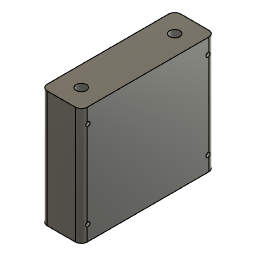
VibrometerPositioningTable v34 (Autodesk Fusion 360 archive; units mm, degrees)
design "Base Spacer"
Autodesk Fusion 360 part; units mm, degrees
sketch "Sketch1" plane through (0, 0, 0) normal (0, 1, 0) x (1, 0, 0)
  line L0 (-12, 40) -> (12, 40)
  line L1 (12, 40) -> (12, -40)
  line L2 (12, -40) -> (-12, -40)
  line L3 (-12, -40) -> (-12, 40)
  line L4 (-50, 0) -> (40, 0) construction
  line L5 (0, 60) -> (0, -56.3927) construction
  circle A0 centre (0, -28) radius 3.1
  circle A1 centre (0, 28) radius 3.1
  dimension "d1" = 24
  dimension "d2" = 80
  dimension "d3" = 12
  dimension "d4" = 40
  dimension "d5" = 6.2
  dimension "d6" = 12
  dimension "d7" = 12
  constraint horizontal L0
  constraint vertical L1
  constraint horizontal L2
  constraint vertical L3
  constraint horizontal L4
  constraint perpendicular L2 L5
  constraint symmetric L4 A0 A1
  measures "d1" distance of L0.start L0.end
  measures "d2" distance of L0.start L2.end
  measures "d3" distance of L3 L5
  measures "d4" distance of L0 L4
  measures "d5" diameter of A0
  measures "d6" distance of L3 A0.centre
  measures "d7" distance of L2 A0.centre
extrude "Extrude1" add sketch "Sketch1" along normal blind 70
fillet "Fillet1" radius 3.5 4 edges at (-12, 35, 40) (-12, 35, -40) (12, 35, -40) (12, 35, 40)
sketch "Sketch3" plane through (12, 0, 0) normal (1, 0, 0) x (0, 0, -1)
  line L0 (-36.5, 70) -> (-36.5, 0)
  line L1 (-36.5, 0) -> (36.5, 0)
  line L2 (36.5, 0) -> (36.5, 70)
  line L3 (36.5, 70) -> (-36.5, 70)
  line L4 (36, 9) -> (-36, 9)
  line L5 (-36, 9) -> (-36, 61)
  line L6 (-36, 61) -> (36, 61)
  line L7 (36, 61) -> (36, 9)
  line L8 (36, 9) -> (-36, 61) construction
  line L9 (-36, 9) -> (36, 61) construction
  circle A0 centre (-36, 61) radius 1.25
  circle A1 centre (36, 61) radius 1.25
  circle A2 centre (-36, 9) radius 1.25
  circle A3 centre (36, 9) radius 1.25
  point P0 (0, 35)
  dimension "d12" = 72
  dimension "d13" = 52
  dimension "d14" = 36.5
  dimension "d15" = 73
  dimension "d16" = 2.5
  dimension "d17" = 2.5
  dimension "d18" = 2.5
  dimension "d19" = 2.5
  dimension "d20" = 70
  dimension "d21" = 35
  constraint horizontal L4
  constraint perpendicular L4 L5
  constraint parallel L4 L6
  constraint parallel L5 L7
  constraint coincident L8 P0
  constraint coincident L9 P0
  constraint coincident L5.end L6.start
  constraint coincident L6.end L7.start
  constraint coincident L4.end L5.start
  constraint coincident L4.start L7.end
  measures "d12" distance of L5.end L6.end
  measures "d13" distance of L4.end L5.end
  measures "d14" distance of L0 P0
  measures "d15" distance of L0.start L2.end
  measures "d16" diameter of A0
  measures "d17" diameter of A1
  measures "d18" diameter of A2
  measures "d19" diameter of A3
  measures "d20" distance of L1 L3
  measures "d21" distance of L3 P0
extrude "Extrude2" cut sketch "Sketch3" against normal blind 24 contours L0 L5 L6 A0 | L0 A0 | L5 L6 A0 | L2 A1 | L2 L6 L7 A1 | L0 L4 L5 A2 | L0 A2 | L6 L7 A1 | L4 L5 A2 | L2 A3 | L2 L4 L7 A3 | L4 L7 A3
equation "d3 = d1 / 2"
equation "d4 = d2 / 2"
equation "d7 = d6"
equation "d14 = d15 / 2"
equation "d17 = d16"
equation "d18 = d16"
equation "d19 = d16"
equation "d21 = d20 / 2"

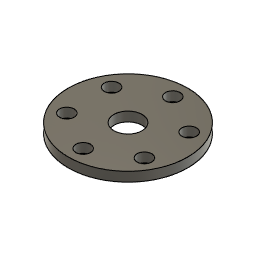
design "HubSpacer2"
Autodesk Fusion 360 part; units mm, degrees
sketch "Sketch1" plane through (0, 0, 0) normal (0, 1, 0) x (1, 0, 0)
  circle A0 centre (0, 0) radius 12.7
  circle A1 centre (0, 0) radius 9.525 construction
  circle A2 centre (-0.0005, 9.525) radius 1.55
  circle A3 centre (-8.2491, 4.7621) radius 1.55
  circle A4 centre (-8.2487, -4.7629) radius 1.55
  circle A5 centre (0.0005, -9.525) radius 1.55
  circle A6 centre (8.2491, -4.7621) radius 1.55
  circle A7 centre (8.2487, 4.7629) radius 1.55
  circle A8 centre (0, 0) radius 3
  dimension "d1" = 25.4
  dimension "d2" = 19.05
  dimension "d3" = 3.1
  dimension "d5" = 360
  dimension "d6" = 6
  constraint coincident A0.centre A1.centre
  constraint concentric A0 A1
  constraint coincident A1 A2.centre
  measures "d1" diameter of A0
  measures "d2" diameter of A1
  measures "d3" diameter of A2
  measures "d6" diameter of A8
extrude "Extrude1" add sketch "Sketch1" along normal blind 2

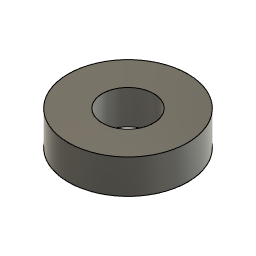
design "BallBearing12x28x8"
Autodesk Fusion 360 part; units mm, degrees
sketch "Sketch1" plane through (0, 0, 0) normal (0, 1, 0) x (1, 0, 0)
  circle A0 centre (0, 0) radius 6
  circle A1 centre (0, 0) radius 14
  dimension "d1" = 12
  dimension "d2" = 28
  constraint coincident A0.centre A1.centre
  constraint concentric A0 A1
  measures "d1" diameter of A0
  measures "d2" diameter of A1
extrude "Extrude1" add sketch "Sketch1" along normal blind 8

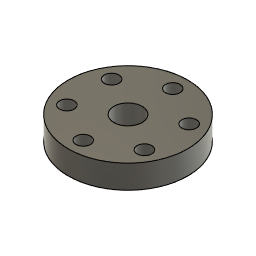
design "HubSpacer5"
Autodesk Fusion 360 part; units mm, degrees
sketch "Sketch1" plane through (0, 0, 0) normal (0, 1, 0) x (1, 0, 0)
  circle A0 centre (0, 0) radius 12.7
  circle A1 centre (0, 0) radius 9.525 construction
  circle A2 centre (-0.0005, 9.525) radius 1.55
  circle A3 centre (-8.2491, 4.7621) radius 1.55
  circle A4 centre (-8.2487, -4.7629) radius 1.55
  circle A5 centre (0.0005, -9.525) radius 1.55
  circle A6 centre (8.2491, -4.7621) radius 1.55
  circle A7 centre (8.2487, 4.7629) radius 1.55
  circle A8 centre (0, 0) radius 3
  dimension "d1" = 25.4
  dimension "d2" = 19.05
  dimension "d3" = 3.1
  dimension "d5" = 360
  dimension "d6" = 6
  constraint coincident A0.centre A1.centre
  constraint concentric A0 A1
  constraint coincident A1 A2.centre
  measures "d1" diameter of A0
  measures "d2" diameter of A1
  measures "d3" diameter of A2
  measures "d6" diameter of A8
extrude "Extrude1" add sketch "Sketch1" along normal blind 5

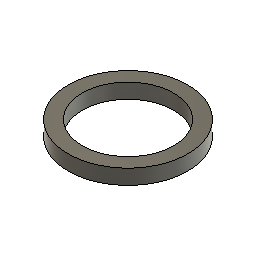
design "BallBearing55x72x9"
Autodesk Fusion 360 part; units mm, degrees
sketch "Sketch1" plane through (0, 0, 0) normal (0, 1, 0) x (1, 0, 0)
  circle A0 centre (0, 0) radius 27.5
  circle A1 centre (0, 0) radius 36
  dimension "d1" = 55
  dimension "d2" = 72
  constraint coincident A0.centre A1.centre
  constraint concentric A0 A1
  measures "d1" diameter of A0
  measures "d2" diameter of A1
extrude "Extrude1" add sketch "Sketch1" along normal blind 9

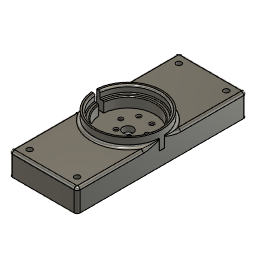
design "StaticBase"
Autodesk Fusion 360 part; units mm, degrees
sketch "Sketch1" plane through (0, 0, 0) normal (0, 1, 0) x (-1, 0, 0)
  circle A0 centre (7.75, 53.037581) radius 1.5
  circle A1 centre (7.75, 26.190794) radius 1.5
  circle A2 centre (-15.5, 39.614187) radius 1.5
  circle A3 centre (-7.75, 26.190794) radius 1.5
  circle A4 centre (15.5, 39.614187) radius 1.5
  circle A5 centre (-7.75, 53.037581) radius 1.5
  circle A6 centre (0, 46.614187) radius 6
  circle A7 centre (-15.5, 39.614187) radius 1.6
  circle A8 centre (-7.75, 53.037581) radius 1.6
  circle A9 centre (7.75, 53.037581) radius 1.6
  circle A10 centre (15.5, 39.614187) radius 1.6
  circle A11 centre (7.75, 26.190794) radius 1.6
  circle A12 centre (-7.75, 26.190794) radius 1.6
  circle A13 centre (0, 46.614187) radius 6.15
  line L0 (40, 39.614187) -> (40, 146.614187)
  line L1 (-40, 39.614187) -> (-40, 146.614187)
  line L2 (-40, 39.614187) -> (-40, -53.385813)
  line L3 (-40, -53.385813) -> (40, -53.385813)
  line L4 (40, -53.385813) -> (40, 39.614187)
  line L5 (40, 146.614187) -> (-40, 146.614187)
  line L6 (40, -13.385813) -> (-40, -13.385813)
  line L7 (40, 106.614187) -> (-40, 106.614187)
  line L8 (0, 150) -> (0, -80) construction
  line L9 (46.540026, 46.614187) -> (-48.931314, 46.614187) construction
  circle A14 centre (0, 39.614187) radius 15.5
  line L10 (35, -13.385813) -> (35, 106.614187)
  line L11 (-35, -13.385813) -> (-35, 106.614187)
  dimension "d24" = 40
  dimension "d25" = 40
  dimension "d5" = 100
  dimension "d6" = 100
  dimension "d11" = 12.3
  dimension "d12" = 3.2
  dimension "d13" = 3.2
  dimension "d14" = 3.2
  dimension "d15" = 3.2
  dimension "d16" = 3.2
  dimension "d17" = 3.2
  dimension "d18" = 15.5
  dimension "d19" = 7
  dimension "d28" = 31
  dimension "d29" = 7
  dimension "d31" = 40
  dimension "d32" = 40
  dimension "d35" = 5
  dimension "d36" = 5
  constraint concentric A5 A8
  constraint concentric A0 A9
  constraint concentric A1 A11
  constraint concentric A3 A12
  constraint concentric A6 A13
  constraint vertical L0
  constraint vertical L1
  constraint perpendicular L0 L3
  constraint perpendicular L3 L4
  constraint perpendicular L0 L5
  constraint perpendicular L2 L6
  constraint perpendicular L1 L7
  constraint perpendicular L5 L8
  constraint perpendicular L1 L9
  constraint symmetric A7 A10 L8
  constraint perpendicular L7 L10
  constraint perpendicular L7 L11
  measures "d24" distance of L3 L6
  measures "d25" distance of L5 L7
  measures "d5" distance of L3 L9
  measures "d6" distance of L5 L9
  measures "d11" diameter of A13
  measures "d12" diameter of A9
  measures "d13" diameter of A10
  measures "d14" diameter of A11
  measures "d15" diameter of A12
  measures "d16" diameter of A7
  measures "d17" diameter of A8
  measures "d28" diameter of A14
  measures "d31" distance of L4 L8
  measures "d32" distance of L2 L8
  measures "d35" distance of L0 L10
  measures "d36" distance of L1 L11
extrude "Extrude7" add sketch "Sketch1" along normal blind 6.5 contours A7 A8 A9 A10 A11 A12 A14 | L0 L4 L6 L7 L10 | L0 L1 L5 L7 | L2 L3 L4 L6 | L6 L7 L10 L11 | L1 L2 L6 L7 L11 picked at (7.996831, 33.64073) picked at (36.666667, 44.280854) picked at (-11.666667, 133.280854) picked at (-11.666667, -40.052479) picked at (0, 89.447521) picked at (-36.666667, 44.280854)
extrude "Extrude8" add sketch "Sketch1" against normal blind 10 contours L0 L4 L6 L7 L10 | L0 L1 L5 L7 | L2 L3 L4 L6 | L1 L2 L6 L7 L11 picked at (36.666667, 44.280854) picked at (-11.666667, 133.280854) picked at (-11.666667, -40.052479) picked at (-36.666667, 44.280854)
sketch "Sketch3" plane through (0, 6.5, 0) normal (0, 1, 0) x (-1, 0, 0)
  circle A0 centre (7.75, 26.190794) radius 1.6
  circle A1 centre (15.5, 39.614187) radius 1.6
  circle A2 centre (0, 46.614187) radius 6.15
  circle A3 centre (7.75, 53.037581) radius 1.6
  circle A4 centre (-7.75, 26.190794) radius 1.6
  circle A5 centre (-15.5, 39.614187) radius 1.6
  circle A6 centre (-7.75, 53.037581) radius 1.6
  line L0 (-40, 146.614187) -> (-40, -53.385813)
  line L1 (-40, -53.385813) -> (40, -53.385813)
  line L2 (40, -53.385813) -> (40, 146.614187)
  line L3 (40, 146.614187) -> (-40, 146.614187)
  circle A7 centre (0, 46.614187) radius 31.75
  circle A8 centre (0, 46.614187) radius 40
  line L4 (31.75, 46.614187) -> (40, 46.614187) construction
  line L5 (31.60795, 49.614187) -> (39.887341, 49.614187)
  line L6 (31.60795, 43.614187) -> (39.887341, 43.614187)
  dimension "d39" = 63.5
  dimension "d41" = 3
  constraint concentric A2 A7
  constraint concentric A7 A8
  constraint tangent L2 A8
  constraint perpendicular L2 L4
  constraint perpendicular L2 L5
  measures "d39" diameter of A7
  measures "d41" distance of L4 L5
extrude "Extrude9" add sketch "Sketch3" along normal blind 12 contours A7 A8 L5 L6 picked at (-37.078885, 43.888312)
sketch "Sketch4" plane through (0, 18.5, 0) normal (0, 1, 0) x (-1, 0, 0)
  line L0 (31.60795, 49.614187) -> (39.887341, 49.614187)
  arc A0 (39.887341, 49.614187) -> (39.887341, 43.614187) centre (0, 46.614187) ccw
  line L1 (39.887341, 43.614187) -> (31.60795, 43.614187)
  arc A1 (31.60795, 49.614187) -> (31.60795, 43.614187) centre (0, 46.614187) ccw
  circle A2 centre (0, 46.614187) radius 36.15
  dimension "d44" = 72.3
  constraint concentric A0 A2
  measures "d44" diameter of A2
extrude "Extrude10" add sketch "Sketch4" along normal blind 8.5 contours L0 A0 L1 A2 picked at (38.30249, 51.58448)
fillet "Fillet6" radius 1 6 edges at (16.991724, 6.5, 40.192772) (9.241724, 6.5, 53.616166) (9.241724, 6.5, 26.769378) (-6.258276, 6.5, 26.769378) (-14.008276, 6.5, 40.192772) (-6.258276, 6.5, 53.616166)
fillet "Fillet7" radius 1 2 edges at (31.75, 18.5, 46.614187) (36.15, 18.5, 46.614187)
fillet "Fillet8" radius 2 1 edges at (36.15, 27, 46.614187)
sketch "Sketch5" plane through (0, 6.5, 0) normal (0, 1, 0) x (-1, 0, 0)
  line L0 (40, -53.385813) -> (40, 146.614187)
  line L1 (40, 146.614187) -> (-40, 146.614187)
  line L2 (-40, 146.614187) -> (-40, 46.614187)
  circle A0 centre (28, 134.614187) radius 3.1
  line L3 (0, 160.139832) -> (0, -64.91971) construction
  line L4 (38.031862, 43.614187) -> (36.025304, 43.614187)
  line L5 (36.025304, 49.614187) -> (38.031862, 49.614187)
  line L6 (42.850808, 46.614187) -> (-49.000001, 46.614187) construction
  line L7 (35.021743, 43.614187) -> (32.612306, 43.614187)
  line L8 (32.612306, 49.614187) -> (35.021743, 49.614187)
  circle A1 centre (-7.75, 53.037581) radius 1.6
  circle A2 centre (7.75, 53.037581) radius 1.6
  circle A3 centre (-28, 134.614187) radius 3.1
  circle A4 centre (-28, -41.385813) radius 3.1
  circle A5 centre (28, -41.385813) radius 3.1
  circle A6 centre (15.5, 39.614187) radius 2.6
  circle A7 centre (-7.75, 26.190794) radius 2.6
  circle A8 centre (-15.5, 39.614187) radius 2.6
  arc A9 (39.887341, 49.614187) -> (-40, 46.614187) centre (0, 46.614187) ccw
  line L9 (39.887341, 49.614187) -> (31.60795, 49.614187)
  arc A10 (31.60795, 49.614187) -> (31.60795, 43.614187) centre (0, 46.614187) ccw
  line L10 (31.60795, 43.614187) -> (39.887341, 43.614187)
  arc A11 (-40, 46.614187) -> (39.887341, 43.614187) centre (0, 46.614187) ccw
  line L11 (-40, 46.614187) -> (-40, -53.385813)
  line L12 (-40, -53.385813) -> (40, -53.385813)
  circle A12 centre (0, 46.614187) radius 6.15
  circle A13 centre (-7.75, 53.037581) radius 2.6
  circle A14 centre (7.75, 26.190794) radius 2.6
  circle A15 centre (7.75, 53.037581) radius 2.6
  circle A16 centre (0, 46.614187) radius 40
  line L13 (39.887341, 43.614187) -> (40, 43.614187)
  line L14 (39.887341, 49.614187) -> (40, 49.614187)
  line L15 (-39.887341, 43.614187) -> (-40, 43.614187)
  line L16 (-39.887341, 49.614187) -> (-40, 49.614187)
  dimension "d55" = 6.2
  dimension "d56" = 12
  dimension "d57" = 12
  dimension "d60" = 3
  dimension "d62" = 6
  dimension "d63" = 3.2
  dimension "d64" = 3.2
  dimension "d65" = 15.5
  dimension "d66" = 7.75
  constraint perpendicular L1 L3
  constraint horizontal L6
  constraint symmetric A0 L3 A3
  constraint symmetric A0 L6 A5
  constraint symmetric L6 A3 A4
  constraint concentric A9 A16
  constraint perpendicular L0 L13
  measures "d55" diameter of A0
  measures "d60" distance of L6 L7
  measures "d62" distance of L7 L8
  measures "d63" diameter of A1
  measures "d64" diameter of A2
extrude "Extrude11" cut sketch "Sketch5" against normal blind 16.5 contours A0 | A3 | A4 | A5 picked at (27.483333, 132.822601) picked at (-28.516667, 132.822601) picked at (-29.390878, -41.834159) picked at (26.609122, -41.834159)
extrude "Extrude12" add sketch "Sketch5" along normal blind 10 contours L0 A11 L11 L12 A16 L13 L15 | L0 L1 L2 A9 A16 L14 L16 picked at (0, -24.221618) picked at (0, 117.449993)
fillet "Fillet9" radius 3.5 4 edges at (40, 3.25, 146.614187) (-40, 3.25, 146.614187) (40, 3.25, -53.385813) (-40, 3.25, -53.385813)
fillet "Fillet10" radius 3 12 edges at (0, 16.5, 6.614187) (0, 16.5, 86.614187) (-40, 16.5, 96.364187) (-38.974874, 16.5, 145.589061) (0, 16.5, 146.614187) (38.974874, 16.5, 145.589061) (40, 16.5, 96.364187) (40, 16.5, -3.135813) (38.974874, 16.5, -52.360686) (0, 16.5, -53.385813) (-38.974874, 16.5, -52.360686) (-40, 16.5, -3.135813)
equation "d25 = d24"
equation "d6 = d5"
equation "d13 = d12"
equation "d14 = d12"
equation "d15 = d12"
equation "d16 = d12"
equation "d17 = d12"
equation "d32 = d31"
equation "d36 = d35"
equation "d39 = ( ( 72 - 55 ) / 2 ) * 1 mm + 55 mm"
equation "d56 = ( d55 - 0.2 mm ) * 2"
equation "d57 = d56"
equation "d66 = d65 / 2"

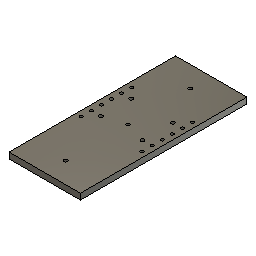
design "plywood_plate"
Autodesk Fusion 360 part; units mm, degrees
sketch "Sketch1" plane through (0, 0, 0) normal (0, 1, 0) x (1, 0, 0)
  line L0 (60, 140) -> (-60, 140)
  line L1 (-60, 140) -> (-60, -140)
  line L2 (-60, -140) -> (60, -140)
  line L3 (60, -140) -> (60, 140)
  line L4 (60, 140) -> (-60, -140) construction
  line L5 (-60, 140) -> (60, -140) construction
  line L6 (0, 160) -> (0, -180) construction
  line L7 (-113.0657, 15) -> (80.2615, 15) construction
  line L8 (80.2615, 15) -> (130.9595, 14.8382) construction
  line L9 (130.9595, 14.8382) -> (130.9763, 20.0945) construction
  line L10 (130.9763, 20.0945) -> (80.2783, 20.2563) construction
  line L11 (80.2783, 20.2563) -> (80.2615, 15) construction
  circle A0 centre (0, -105) radius 3
  circle A1 centre (0, 0) radius 3
  line L12 (-100.8455, 0) -> (89.1545, 0) construction
  circle A2 centre (0, 105) radius 3
  circle A3 centre (51, 23.5) radius 2.5
  circle A4 centre (51, 40.5) radius 2.5
  circle A5 centre (51, 57.5) radius 2.5
  line L13 (51, 19.633) -> (51, 57.5)
  line L14 (60, 40.5) -> (35, 40.5)
  circle A6 centre (35, 40.5) radius 3
  circle A7 centre (51, 6.5) radius 2.5
  circle A8 centre (51, -10.5) radius 2.5
  circle A9 centre (51, -27.5) radius 2.5
  circle A10 centre (35, -10.5) radius 3
  circle A11 centre (-35, -10.5) radius 3
  circle A12 centre (-51, -10.5) radius 2.5
  circle A13 centre (-51, 6.5) radius 2.5
  circle A14 centre (-51, 23.5) radius 2.5
  circle A15 centre (-51, 40.5) radius 2.5
  circle A16 centre (-51, 57.5) radius 2.5
  circle A17 centre (-35, 40.5) radius 3
  circle A18 centre (-51, -27.5) radius 2.5
  dimension "d1" = 120
  dimension "d2" = 280
  dimension "d3" = 5
  dimension "d4" = 155
  dimension "d5" = 6
  dimension "d6" = 35
  dimension "d7" = 6
  dimension "d11" = 5
  dimension "d12" = 9
  dimension "d14" = 5
  dimension "d15" = 17
  dimension "d16" = 5
  dimension "d17" = 17
  dimension "d18" = 25
  dimension "d19" = 6
  dimension "d20" = 8.5
  dimension "d21" = 15
  constraint horizontal L0
  constraint perpendicular L0 L1
  constraint parallel L0 L2
  constraint parallel L1 L3
  constraint coincident L4 A1.centre
  constraint coincident L5 A1.centre
  constraint coincident A1.centre origin
  constraint perpendicular L2 L6
  constraint coincident L7.end
  constraint coincident L6 A0.centre
  constraint coincident L6 A1.centre
  constraint perpendicular L3 L12
  constraint coincident A1.centre L12
  constraint coincident A1.centre L6
  constraint symmetric A0 L12 A2
  constraint coincident A5.centre L13.end
  constraint coincident A3.centre L13
  constraint coincident A4.centre L13
  constraint coincident L3 L14.start
  constraint perpendicular L3 L14
  constraint coincident L14.end A6.centre
  constraint coincident A4.centre L14
  constraint perpendicular L7 L13
  constraint symmetric L7 A3 A7
  constraint symmetric L7 A4 A8
  constraint symmetric L7 A5 A9
  constraint symmetric L7 A6 A10
  constraint symmetric L6 A3 A14
  constraint symmetric L6 A4 A15
  constraint symmetric L6 A5 A16
  constraint symmetric L6 A6 A17
  constraint symmetric L6 A7 A13
  constraint symmetric L6 A8 A12
  constraint symmetric L6 A10 A11
  constraint symmetric L6 A9 A18
  measures "d1" distance of L1.end L2.end
  measures "d2" distance of L0.end L1.end
  measures "d4" distance of L2 L7
  measures "d5" diameter of A0
  measures "d6" distance of L2 A0.centre
  measures "d7" diameter of A1
  measures "d11" diameter of A3
  measures "d12" distance of L3 A3.centre
  measures "d14" diameter of A4
  measures "d15" distance of A3.centre A4.centre
  measures "d16" diameter of A5
  measures "d17" distance of A4.centre A5.centre
  measures "d18" distance of L14.start L14.end
  measures "d19" diameter of A6
  measures "d20" distance of L7 A3.centre
  measures "d21" distance of L7 L12
extrude "Extrude1" add sketch "Sketch1" along normal blind 10
equation "d18 = 22.00 mm + ( d19 / 2 mm ) * 1 mm"

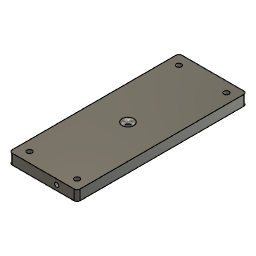
design "Down Table"
Autodesk Fusion 360 part; units mm, degrees
sketch "Sketch1" plane through (0, 0, 0) normal (0, 1, 0) x (1, 0, 0)
  line L0 (0, 130) -> (0, -122.2085) construction
  line L1 (-100, 0) -> (125, 0) construction
  line L2 (40, 100) -> (-40, 100)
  line L3 (-40, 100) -> (-40, -100)
  line L4 (-40, -100) -> (40, -100)
  line L5 (40, -100) -> (40, 100)
  line L6 (40, 100) -> (-40, -100) construction
  line L7 (-40, 100) -> (40, -100) construction
  circle A0 centre (-28, -88) radius 3
  circle A1 centre (0, 0) radius 3
  circle A2 centre (-28, 88) radius 3
  circle A3 centre (28, 88) radius 3
  circle A4 centre (28, -88) radius 3
  dimension "d1" = 80
  dimension "d2" = 200
  dimension "d3" = 6
  dimension "d4" = 6
  dimension "d5" = 12
  dimension "d6" = 12
  constraint vertical L0
  constraint horizontal L1
  constraint horizontal L2
  constraint perpendicular L2 L3
  constraint parallel L2 L4
  constraint parallel L3 L5
  constraint coincident L6 A1.centre
  constraint coincident L7 A1.centre
  constraint coincident A1.centre origin
  constraint symmetric L1 A0 A2
  constraint symmetric L0 A0 A4
  constraint symmetric L0 A2 A3
  measures "d1" distance of L3.end L4.end
  measures "d2" distance of L2.end L3.end
  measures "d3" diameter of A0
  measures "d4" diameter of A1
  measures "d5" distance of L4 A0.centre
  measures "d6" distance of L3 A0.centre
extrude "Extrude1" add sketch "Sketch1" along normal blind 12
fillet "Fillet1" radius 4 1 edges at (-2.797, 12, -1.0848)
fillet "Fillet2" radius 3.5 4 edges at (40, 6, -100) (-40, 6, -100) (-40, 6, 100) (40, 6, 100)
sketch "Sketch2" plane through (0, 0, 100) normal (0, 0, 1) x (1, 0, 0)
  line L0 (36.5, 0) -> (36.5, 12)
  line L1 (36.5, 12) -> (-36.5, 12)
  line L2 (-36.5, 12) -> (-36.5, 0)
  line L3 (-36.5, 0) -> (36.5, 0)
  line L4 (0, 12) -> (0, 0) construction
  line L5 (7, 12) -> (7, 0) construction
  line L6 (7, 12) -> (-7, 12) construction
  line L7 (25, 12) -> (31, 12) construction
  line L8 (25, 12) -> (25, 0) construction
  line L9 (25, 0) -> (7, 12) construction
  line L10 (7, 0) -> (25, 12) construction
  circle A0 centre (16, 6) radius 2.5
  dimension "d13" = 7
  dimension "d14" = 14
  dimension "d15" = 6
  dimension "d16" = 5
  constraint midpoint L1 L4.start
  constraint coincident L4.end origin
  constraint coincident L1 L5.start
  constraint coincident L3 L5.end
  constraint perpendicular L3 L5
  constraint coincident L7.start L8.start
  constraint coincident L3 L8.end
  constraint perpendicular L3 L8
  constraint midpoint L9 A0.centre
  measures "d13" distance of L4 L5
  measures "d14" distance of L5.start L6.end
  measures "d15" distance of L7.start L7.end
  measures "d16" diameter of A0
extrude "Extrude2" cut sketch "Sketch2" against normal blind 200 contours A0
equation "d6 = d5"
equation "d13 = d14 / 2"

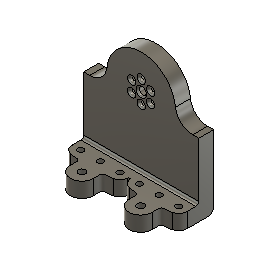
design "HolderBase"
Autodesk Fusion 360 part; units mm, degrees
sketch "Sketch1" plane through (0, 20, -46.4489) normal (0, 0, 1) x (-1, 0, 0)
  circle A0 centre (0.9947, -83.8573) radius 3
  circle A1 centre (0.9947, -83.8573) radius 6
  circle A2 centre (0.9947, -83.8573) radius 6
  circle A3 centre (0.9947, -83.8573) radius 3.05
  circle A4 centre (0.9947, -83.8573) radius 30
  line L0 (50.9947, -10.8573) -> (-49.0053, -10.8573)
  line L1 (-49.0053, -10.8573) -> (-49.0053, -83.8573)
  line L2 (-49.0053, -83.8573) -> (50.9947, -83.8573)
  line L3 (50.9947, -83.8573) -> (50.9947, -10.8573)
  line L4 (50.9947, -10.8573) -> (-49.0053, -83.8573) construction
  line L5 (-49.0053, -10.8573) -> (50.9947, -83.8573) construction
  line L6 (-49.0053, -23.8573) -> (50.9947, -23.8573)
  line L7 (-49.0053, -73.8573) -> (50.9947, -73.8573)
  point P0 (0.9947, -47.3573)
  dimension "d70" = 60
  dimension "d111" = 12
  dimension "d208" = 50
  dimension "d209" = 100
  dimension "d210" = 13
  dimension "d6" = 6.1
  dimension "d18" = 60
  dimension "d19" = 10
  constraint concentric A0 A2
  constraint concentric A2 A3
  constraint concentric A2 A4
  constraint horizontal L0
  constraint perpendicular L0 L1
  constraint parallel L0 L2
  constraint parallel L1 L3
  constraint coincident L4 P0
  constraint coincident L5 P0
  constraint coincident A0.centre L2
  constraint coincident L1 L6.start
  constraint coincident L3 L6.end
  constraint perpendicular L3 L6
  constraint coincident L1 L7.start
  constraint coincident L3 L7.end
  constraint perpendicular L3 L7
  measures "d70" diameter of A4
  measures "d111" diameter of A2
  measures "d208" distance of A0.centre L1
  measures "d209" distance of L0.start L0.end
  measures "d210" distance of L0 L6
  measures "d6" diameter of A3
  measures "d18" distance of L2 L6
  measures "d19" distance of L2 L7
extrude "Extrude1" add sketch "Sketch1" along normal blind 13 contours A1 A2 A3 L2 | A1 A2 A3 L2 | A1 A2 A4 L2 | A1 A2 A4 L2 L7 | A4 L7 | A4 L1 L3 L6 L7
extrude "Extrude6" add sketch "Sketch1" along normal blind 53 contours L0 L1 L3 L6
sketch "Sketch2" plane through (0, 43.8573, 0) normal (0, 1, 0) x (-1, 0, 0)
  line L0 (-49.0053, -33.4489) -> (50.9947, -33.4489)
  line L1 (50.9947, -33.4489) -> (50.9947, 6.5511)
  line L2 (50.9947, 6.5511) -> (-49.0053, 6.5511)
  line L3 (-49.0053, 6.5511) -> (-49.0053, -33.4489)
  line L4 (0.9947, -100) -> (0.9947, 25)
  circle A0 centre (43.4947, -23.4489) radius 2.55
  circle A1 centre (43.4947, -23.4489) radius 7.5
  line L5 (50.9947, -33.4489) -> (-49.0053, -33.4489)
  line L6 (-49.0053, -33.4489) -> (-49.0053, 6.5511)
  line L7 (-49.0053, 6.5511) -> (50.9947, 6.5511)
  line L8 (50.9947, 6.5511) -> (50.9947, -33.4489)
  circle A2 centre (26.4947, -23.4489) radius 7.5
  circle A3 centre (26.4947, -23.4489) radius 2.55
  circle A4 centre (9.4947, -23.4489) radius 7.5
  circle A5 centre (9.4947, -23.4489) radius 2.55
  line L9 (50.9947, -23.4489) -> (0.9947, -23.4489)
  circle A6 centre (-41.5053, -23.4489) radius 7.5
  circle A7 centre (-41.5053, -23.4489) radius 2.55
  line L10 (-49.0053, -23.4489) -> (0.9947, -23.4489)
  circle A8 centre (-24.5053, -23.4489) radius 7.5
  circle A9 centre (-24.5053, -23.4489) radius 2.55
  circle A10 centre (-7.5053, -23.4489) radius 7.5
  circle A11 centre (-7.5053, -23.4489) radius 2.55
  circle A12 centre (26.4947, -7.4489) radius 3.05
  circle A13 centre (26.4947, -7.4489) radius 10
  line L11 (50.9947, -7.4489) -> (0.9947, -7.4489)
  spline S0 degree 5 poles (36.4947, -7.4489) (36.5142, -7.782) (36.5365, -8.4586) (36.5197, -9.5049) (36.4281, -10.9328) (36.3682, -12.6126) (36.5621, -14.004) (37.1816, -14.9597) (38.3015, -15.4385) (39.8392, -15.5688) (41.6323, -15.5639) (43.1209, -15.6414) (44.1969, -15.8336) (44.8868, -16.0334) (45.2248, -16.1512) knots 0 0 0 0 0 0 0.1 0.2 0.3 0.4 0.5 0.6 0.7 0.8 0.9 1 1 1 1 1 1
  line L12 (26.4947, -23.4489) -> (26.4947, -7.4489) construction
  spline S1 degree 5 poles (16.4947, -7.4489) (16.4752, -7.782) (16.453, -8.4586) (16.4698, -9.5049) (16.5613, -10.9328) (16.6213, -12.6126) (16.4274, -14.004) (15.8079, -14.9597) (14.688, -15.4385) (13.1502, -15.5688) (11.3571, -15.5639) (9.8686, -15.6414) (8.7925, -15.8336) (8.1027, -16.0334) (7.7647, -16.1512) knots 0 0 0 0 0 0 0.1 0.2 0.3 0.4 0.5 0.6 0.7 0.8 0.9 1 1 1 1 1 1
  line L13 (36.3896, -5.6527) -> (36.5999, -9.2451)
  line L14 (43.5142, -15.5551) -> (46.9353, -16.7473)
  line L15 (16.5999, -5.6527) -> (16.3896, -9.2451)
  line L16 (9.4753, -15.5551) -> (6.0541, -16.7473)
  circle A14 centre (-24.5053, -7.4489) radius 10
  circle A15 centre (-24.5053, -7.4489) radius 3.05
  line L17 (-49.0053, -7.4489) -> (0.9947, -7.4489)
  spline S2 degree 5 poles (-14.5053, -7.4489) (-14.4858, -7.782) (-14.4635, -8.4586) (-14.4803, -9.5049) (-14.5719, -10.9328) (-14.6318, -12.6126) (-14.4379, -14.004) (-13.8184, -14.9597) (-12.6985, -15.4385) (-11.1608, -15.5688) (-9.3677, -15.5639) (-7.8791, -15.6414) (-6.8031, -15.8336) (-6.1132, -16.0334) (-5.7752, -16.1512) knots 0 0 0 0 0 0 0.1 0.2 0.3 0.4 0.5 0.6 0.7 0.8 0.9 1 1 1 1 1 1
  line L18 (-14.6104, -5.6527) -> (-14.4001, -9.2451)
  line L19 (-7.4858, -15.5551) -> (-4.0647, -16.7473)
  spline S3 degree 5 poles (-34.5053, -7.4489) (-34.5248, -7.782) (-34.547, -8.4586) (-34.5302, -9.5049) (-34.4387, -10.9328) (-34.3787, -12.6126) (-34.5726, -14.004) (-35.1921, -14.9597) (-36.312, -15.4385) (-37.8498, -15.5688) (-39.6429, -15.5639) (-41.1314, -15.6414) (-42.2075, -15.8336) (-42.8973, -16.0334) (-43.2353, -16.1512) knots 0 0 0 0 0 0 0.1 0.2 0.3 0.4 0.5 0.6 0.7 0.8 0.9 1 1 1 1 1 1
  line L20 (-34.4001, -5.6527) -> (-34.6104, -9.2451)
  line L21 (-41.5247, -15.5551) -> (-44.9459, -16.7473)
  line L22 (45.2248, -16.1512) -> (36.4947, -7.4489) construction
  line L23 (40.8598, -11.8001) -> (26.4947, -23.4489) construction
  point P0 (0.9947, -46.4489)
  point P1 (37.2113, -14.7587)
  point P2 (15.7782, -14.7587)
  point P3 (-13.7887, -14.7587)
  point P4 (-35.2218, -14.7587)
  dimension "d232" = 5.1
  dimension "d233" = 15
  dimension "d234" = 10
  dimension "d237" = -34
  dimension "d238" = 0
  dimension "d239" = 6.1
  dimension "d240" = 20
  dimension "d241" = 16
  constraint perpendicular L2 L4
  constraint coincident L4 P0
  constraint concentric A0 A1
  constraint horizontal L5
  constraint vertical L6
  constraint horizontal L7
  constraint vertical L8
  constraint coincident L2.end L3.start
  constraint coincident L0.end L1.start
  constraint tangent A1 L8
  constraint coincident L8 L9.start
  constraint coincident A1 L9.start
  constraint coincident L4 L9.end
  constraint perpendicular L4 L9
  constraint symmetric L4 A0 A7
  constraint symmetric L4 A1 A6
  constraint symmetric L4 A2 A8
  constraint symmetric L4 A3 A9
  constraint symmetric L4 A4 A10
  constraint symmetric L4 A5 A11
  constraint symmetric L4 L9.start L10.start
  constraint symmetric L4 L9.end L10.end
  constraint concentric A12 A13
  constraint coincident L8 L11.start
  constraint coincident L4 L11.end
  constraint perpendicular L4 L11
  constraint coincident A13 S0.start
  constraint coincident L11 S0.start
  constraint coincident A1 S0.end
  constraint coincident A2.centre A3.centre
  constraint coincident A12.centre A13.centre
  constraint perpendicular L11 L12
  constraint midpoint S0.start L13
  constraint midpoint S0.end L14
  constraint symmetric S0.start L12 S1.start
  constraint symmetric P1 L12 P2
  constraint symmetric S0.end L12 S1.end
  constraint symmetric L12 L13.start L15.start
  constraint symmetric L12 L13.end L15.end
  constraint symmetric L12 L14.start L16.start
  constraint symmetric L12 L14.end L16.end
  constraint symmetric L4 A12 A15
  constraint symmetric L4 A13 A14
  constraint symmetric L4 L11.start L17.start
  constraint symmetric L4 L11.end L17.end
  constraint symmetric L4 S0.start S3.start
  constraint symmetric L4 P1 P4
  constraint symmetric L4 S0.end S3.end
  constraint symmetric L4 S1.start S2.start
  constraint symmetric L4 P2 P3
  constraint symmetric L4 S1.end S2.end
  constraint symmetric L4 L13.start L20.start
  constraint symmetric L4 L13.end L20.end
  constraint symmetric L4 L14.start L21.start
  constraint symmetric L4 L14.end L21.end
  constraint symmetric L4 L15.start L18.start
  constraint symmetric L4 L15.end L18.end
  constraint symmetric L4 L16.start L19.start
  constraint symmetric L4 L16.end L19.end
  constraint coincident A12.centre L11
  constraint midpoint L22 L23.start
  constraint coincident P1 L23
  measures "d232" diameter of A0
  measures "d233" diameter of A1
  measures "d234" distance of A0.centre L5
  measures "d239" diameter of A12
  measures "d240" diameter of A13
  measures "d241" distance of L9 L11
extrude "Extrude9" cut sketch "Sketch2" against normal up to surface (13 mm away) contours L3 L6 A6 L17 S3 | L4 L10 A10 L17 S2 | L4 A4 L9 L11 S1 | L2 L3 L4 L6 L7 A14 L17 | A7 L10 | A7 L10 | L1 A1 L8 L11 S0 | L1 L2 L4 L7 L8 A13 L11 | A0 L9 | A0 L9 | A5 L9 | A5 L9 | L10 A11 | L10 A11 | A15 L17 | A15 L17 | L10 A9 | L10 A9 | A12 L11 | A12 L11 | A3 L9 | A3 L9
fillet "Fillet3" radius 1 2 edges at (-1.9947, 37.3573, -23.4489) (0.0053, 37.3573, -23.4489)
fillet "Fillet4" radius 3 6 edges at (43.8827, 30.8573, -24.371) (26.8827, 30.8573, -24.371) (9.8827, 30.8573, -24.371) (-7.1173, 30.8573, -24.371) (-24.1173, 30.8573, -24.371) (-41.1173, 30.8573, -24.371)
fillet "Fillet5" radius 3.5 2 edges at (27.3489, 30.8573, -8.5519) (-23.6511, 30.8573, -8.5519)
sketch "Sketch3" plane through (0, 0, -46.4489) normal (0, 0, -1) x (-1, 0, 0)
  line L0 (-49.0053, 93.8573) -> (-49.0053, 30.8573)
  line L1 (-49.0053, 30.8573) -> (50.9947, 30.8573)
  line L2 (50.9947, 30.8573) -> (50.9947, 93.8573)
  line L3 (50.9947, 93.8573) -> (29.279, 93.8573)
  arc A0 (29.279, 93.8573) -> (-27.2895, 93.8573) centre (0.9947, 103.8573) ccw
  line L4 (-27.2895, 93.8573) -> (-49.0053, 93.8573)
  circle A1 centre (0.9947, 103.8573) radius 9.525 construction
  line L5 (0.9947, 117.0724) -> (0.9947, 116)
  line L6 (0.9947, 116) -> (0.9947, 91) construction
  circle A2 centre (0.9947, 113.3823) radius 1.55
  circle A3 centre (-7.2542, 108.6198) radius 1.55
  circle A4 centre (-7.2542, 99.0948) radius 1.55
  circle A5 centre (0.9947, 94.3323) radius 1.55
  circle A6 centre (9.2436, 99.0948) radius 1.55
  circle A7 centre (9.2436, 108.6198) radius 1.55
  circle A8 centre (0.9947, 103.8573) radius 3.05
  dimension "d8" = 19.05
  dimension "d9" = 3.1
  dimension "d11" = 360
  constraint concentric A1 A8
  constraint vertical L5
  constraint parallel L5 L6
  constraint coincident A0.centre L6
  constraint coincident L6 A2.centre
  constraint coincident A1 A2.centre
  measures "d8" diameter of A1
  measures "d9" diameter of A2
extrude "Extrude10" cut sketch "Sketch3" against normal blind 15 contours A2 | A3 | A4 | A5 | A6 | A7
fillet "Fillet6" radius 2.1 6 edges at (8.6993, 98.5343, -33.4489) (0.4504, 93.7718, -33.4489) (-7.7985, 98.5343, -33.4489) (-7.7985, 108.0593, -33.4489) (0.4504, 112.8218, -33.4489) (8.6993, 108.0593, -33.4489)
fillet "Fillet6" radius 1.5 1 edges at (1.8489, 102.7544, -33.4489)
fillet "Fillet7" radius 15 2 edges at (27.2895, 93.8573, -39.9489) (-29.279, 93.8573, -39.9489)
fillet "Fillet8" radius 2.5 1 edges at (-0.9947, 43.8573, -33.4489)
fillet "Fillet9" radius 5 1 edges at (-0.9947, 30.8573, -46.4489)
equation "d209 = d208 * 2"
equation "d18 = 1 cm + 4 cm + 1 cm"
